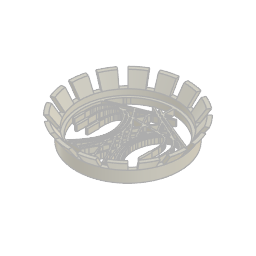
tree-aperture-v10 (Autodesk Fusion 360 design; units mm, degrees)
Autodesk Fusion 360 part; units mm, degrees
(part 1 of 3)
sketch "Sketch1" plane through (0, 0, 0) normal (0, 0, 1) x (1, 0, 0)
  line L0 (24.379, -0.087) -> (23.062, -0.162)
  line L1 (23.062, -0.162) -> (21.745, -0.311)
  line L2 (21.745, -0.311) -> (20.577, -0.509)
  line L3 (20.577, -0.509) -> (19.433, -0.758)
  line L4 (19.433, -0.758) -> (18.067, -1.131)
  line L5 (18.067, -1.131) -> (17.097, -1.454)
  line L6 (17.097, -1.454) -> (16.103, -1.827)
  line L7 (16.103, -1.827) -> (14.886, -2.348)
  line L8 (14.886, -2.348) -> (13.618, -2.97)
  line L9 (13.618, -2.97) -> (12.724, -3.467)
  line L10 (12.724, -3.467) -> (11.705, -4.088)
  line L11 (11.705, -4.088) -> (10.686, -4.784)
  line L12 (10.686, -4.784) -> (9.891, -5.38)
  line L13 (9.891, -5.38) -> (8.574, -6.474)
  line L14 (8.574, -6.474) -> (6.809, -8.188)
  line L15 (6.809, -8.188) -> (5.939, -9.158)
  line L16 (5.939, -9.158) -> (5.244, -10.002)
  line L17 (5.244, -10.002) -> (4.573, -10.897)
  line L18 (4.573, -10.897) -> (3.877, -11.916)
  line L19 (3.877, -11.916) -> (3.231, -12.96)
  line L20 (3.231, -12.96) -> (2.659, -14.003)
  line L21 (2.659, -14.003) -> (2.212, -14.923)
  line L22 (2.212, -14.923) -> (1.764, -15.967)
  line L23 (1.764, -15.967) -> (1.441, -16.812)
  line L24 (1.441, -16.812) -> (0.919, -18.427)
  line L25 (0.919, -18.427) -> (0.547, -19.868)
  line L26 (0.547, -19.868) -> (0.348, -20.862)
  line L27 (0.348, -20.862) -> (0.149, -22.229)
  line L28 (0.149, -22.229) -> (0.025, -23.521)
  line L29 (0.025, -23.521) -> (0, -25.957)
  line L30 (0, -25.957) -> (0.149, -27.87)
  line L31 (0.149, -27.87) -> (0.298, -28.889)
  line L32 (0.298, -28.889) -> (0.596, -30.355)
  line L33 (0.596, -30.355) -> (0.944, -31.672)
  line L34 (0.944, -31.672) -> (1.367, -32.99)
  line L35 (1.367, -32.99) -> (2.137, -34.903)
  line L36 (2.137, -34.903) -> (2.783, -36.22)
  line L37 (2.783, -36.22) -> (3.355, -37.239)
  line L38 (3.355, -37.239) -> (4.647, -39.202)
  line L39 (4.647, -39.202) -> (5.666, -40.519)
  line L40 (5.666, -40.519) -> (6.287, -41.24)
  line L41 (6.287, -41.24) -> (7.828, -42.831)
  line L42 (7.828, -42.831) -> (8.921, -43.8)
  line L43 (8.921, -43.8) -> (10.04, -44.694)
  line L44 (10.04, -44.694) -> (12.003, -46.036)
  line L45 (12.003, -46.036) -> (13.917, -47.13)
  line L46 (13.917, -47.13) -> (15.084, -47.701)
  line L47 (15.084, -47.701) -> (16.327, -48.223)
  line L48 (16.327, -48.223) -> (17.57, -48.67)
  line L49 (17.57, -48.67) -> (18.539, -48.969)
  line L50 (18.539, -48.969) -> (19.906, -49.317)
  line L51 (19.906, -49.317) -> (21.645, -49.64)
  line L52 (21.645, -49.64) -> (21.844, -49.64)
  line L53 (21.844, -49.64) -> (21.993, -49.689)
  line L54 (21.993, -49.689) -> (22.913, -49.789)
  line L55 (22.913, -49.789) -> (24.105, -49.863)
  line L56 (24.105, -49.863) -> (25.323, -49.888)
  line L57 (25.323, -49.888) -> (26.566, -49.838)
  line L58 (26.566, -49.838) -> (28.032, -49.689)
  line L59 (28.032, -49.689) -> (29.125, -49.515)
  line L60 (29.125, -49.515) -> (30.442, -49.242)
  line L61 (30.442, -49.242) -> (31.834, -48.869)
  line L62 (31.834, -48.869) -> (33.052, -48.472)
  line L63 (33.052, -48.472) -> (34.046, -48.099)
  line L64 (34.046, -48.099) -> (35.089, -47.652)
  line L65 (35.089, -47.652) -> (36.158, -47.13)
  line L66 (36.158, -47.13) -> (37.251, -46.533)
  line L67 (37.251, -46.533) -> (38.593, -45.713)
  line L68 (38.593, -45.713) -> (40.383, -44.446)
  line L69 (40.383, -44.446) -> (41.277, -43.725)
  line L70 (41.277, -43.725) -> (42.147, -42.955)
  line L71 (42.147, -42.955) -> (43.067, -42.06)
  line L72 (43.067, -42.06) -> (44.21, -40.793)
  line L73 (44.21, -40.793) -> (44.806, -40.047)
  line L74 (44.806, -40.047) -> (46.123, -38.159)
  line L75 (46.123, -38.159) -> (46.794, -37.04)
  line L76 (46.794, -37.04) -> (47.316, -36.071)
  line L77 (47.316, -36.071) -> (47.763, -35.152)
  line L78 (47.763, -35.152) -> (48.385, -33.685)
  line L79 (48.385, -33.685) -> (48.708, -32.791)
  line L80 (48.708, -32.791) -> (49.155, -31.325)
  line L81 (49.155, -31.325) -> (49.478, -30.007)
  line L82 (49.478, -30.007) -> (49.677, -28.939)
  line L83 (49.677, -28.939) -> (49.925, -26.802)
  line L84 (49.925, -26.802) -> (49.975, -25.882)
  line L85 (49.975, -25.882) -> (49.975, -24.093)
  line L86 (49.975, -24.093) -> (49.801, -22.005)
  line L87 (49.801, -22.005) -> (49.602, -20.738)
  line L88 (49.602, -20.738) -> (49.354, -19.545)
  line L89 (49.354, -19.545) -> (48.981, -18.154)
  line L90 (48.981, -18.154) -> (48.534, -16.787)
  line L91 (48.534, -16.787) -> (48.136, -15.768)
  line L92 (48.136, -15.768) -> (47.689, -14.774)
  line L93 (47.689, -14.774) -> (46.72, -12.935)
  line L94 (46.72, -12.935) -> (45.403, -10.897)
  line L95 (45.403, -10.897) -> (44.483, -9.679)
  line L96 (44.483, -9.679) -> (43.713, -8.76)
  line L97 (43.713, -8.76) -> (42.122, -7.095)
  line L98 (42.122, -7.095) -> (40.905, -6.001)
  line L99 (40.905, -6.001) -> (39.811, -5.132)
  line L100 (39.811, -5.132) -> (38.917, -4.486)
  line L101 (38.917, -4.486) -> (37.898, -3.815)
  line L102 (37.898, -3.815) -> (36.705, -3.119)
  line L103 (36.705, -3.119) -> (35.611, -2.547)
  line L104 (35.611, -2.547) -> (33.673, -1.702)
  line L105 (33.673, -1.702) -> (31.436, -0.957)
  line L106 (31.436, -0.957) -> (30.169, -0.634)
  line L107 (30.169, -0.634) -> (29.175, -0.435)
  line L108 (29.175, -0.435) -> (27.833, -0.236)
  line L109 (27.833, -0.236) -> (26.491, -0.112)
  line L110 (26.491, -0.112) -> (24.379, -0.087)
  line L111 (10.934, -5.529) -> (12.202, -4.66)
  line L112 (12.202, -4.66) -> (12.972, -4.187)
  line L113 (12.972, -4.187) -> (14.14, -3.541)
  line L114 (14.14, -3.541) -> (15.209, -3.019)
  line L115 (15.209, -3.019) -> (17.222, -2.199)
  line L116 (17.222, -2.199) -> (18.191, -1.876)
  line L117 (18.191, -1.876) -> (18.29, -1.876)
  line L118 (18.29, -1.876) -> (18.613, -1.752)
  line L119 (18.613, -1.752) -> (19.831, -1.429)
  line L120 (19.831, -1.429) -> (21.074, -1.18)
  line L121 (21.074, -1.18) -> (22.44, -0.982)
  line L122 (22.44, -0.982) -> (24.503, -0.833)
  line L123 (24.503, -0.833) -> (26.417, -0.857)
  line L124 (26.417, -0.857) -> (26.715, -0.907)
  line L125 (26.715, -0.907) -> (27.361, -0.932)
  line L126 (27.361, -0.932) -> (28.678, -1.106)
  line L127 (28.678, -1.106) -> (29.771, -1.305)
  line L128 (29.771, -1.305) -> (29.871, -1.354)
  line L129 (29.871, -1.354) -> (29.995, -1.354)
  line L130 (29.995, -1.354) -> (30.815, -1.553)
  line L131 (30.815, -1.553) -> (31.933, -1.876)
  line L132 (31.933, -1.876) -> (33.077, -2.274)
  line L133 (33.077, -2.274) -> (34.965, -3.069)
  line L134 (34.965, -3.069) -> (36.332, -3.765)
  line L135 (36.332, -3.765) -> (37.401, -4.386)
  line L136 (37.401, -4.386) -> (38.32, -4.983)
  line L137 (38.32, -4.983) -> (39.389, -5.753)
  line L138 (39.389, -5.753) -> (40.184, -6.374)
  line L139 (40.184, -6.374) -> (41.153, -7.219)
  line L140 (41.153, -7.219) -> (42.893, -8.959)
  line L141 (42.893, -8.959) -> (43.588, -9.754)
  line L142 (43.588, -9.754) -> (44.508, -10.922)
  line L143 (44.508, -10.922) -> (45.452, -12.289)
  line L144 (45.452, -12.289) -> (45.999, -13.183)
  line L145 (45.999, -13.183) -> (46.571, -14.202)
  line L146 (46.571, -14.202) -> (47.068, -15.196)
  line L147 (47.068, -15.196) -> (47.838, -17.035)
  line L148 (47.838, -17.035) -> (48.236, -18.228)
  line L149 (48.236, -18.228) -> (48.559, -19.396)
  line L150 (48.559, -19.396) -> (48.807, -20.49)
  line L151 (48.807, -20.49) -> (49.006, -21.608)
  line L152 (49.006, -21.608) -> (49.13, -22.527)
  line L153 (49.13, -22.527) -> (49.254, -24.267)
  line L154 (49.254, -24.267) -> (49.254, -25.584)
  line L155 (49.254, -25.584) -> (49.205, -26.628)
  line L156 (49.205, -26.628) -> (49.006, -28.467)
  line L157 (49.006, -28.467) -> (48.559, -30.703)
  line L158 (48.559, -30.703) -> (48.236, -31.846)
  line L159 (48.236, -31.846) -> (47.788, -33.164)
  line L160 (47.788, -33.164) -> (46.943, -35.152)
  line L161 (46.943, -35.152) -> (46.248, -36.518)
  line L162 (46.248, -36.518) -> (45.651, -37.537)
  line L163 (45.651, -37.537) -> (44.359, -39.426)
  line L164 (44.359, -39.426) -> (43.539, -40.445)
  line L165 (43.539, -40.445) -> (42.893, -41.166)
  line L166 (42.893, -41.166) -> (42.172, -41.911)
  line L167 (42.172, -41.911) -> (41.153, -42.855)
  line L168 (41.153, -42.855) -> (39.488, -44.197)
  line L169 (39.488, -44.197) -> (39.364, -44.247)
  line L170 (39.364, -44.247) -> (39.165, -44.048)
  line L171 (39.165, -44.048) -> (37.798, -42.458)
  line L172 (37.798, -42.458) -> (36.481, -40.842)
  line L173 (36.481, -40.842) -> (35.065, -38.904)
  line L174 (35.065, -38.904) -> (33.847, -37.09)
  line L175 (33.847, -37.09) -> (33.151, -35.922)
  line L176 (33.151, -35.922) -> (32.43, -34.53)
  line L177 (32.43, -34.53) -> (31.884, -33.213)
  line L178 (31.884, -33.213) -> (31.486, -31.971)
  line L179 (31.486, -31.971) -> (31.238, -30.902)
  line L180 (31.238, -30.902) -> (31.088, -29.908)
  line L181 (31.088, -29.908) -> (30.989, -28.442)
  line L182 (30.989, -28.442) -> (31.039, -26.951)
  line L183 (31.039, -26.951) -> (31.163, -25.932)
  line L184 (31.163, -25.932) -> (31.486, -24.317)
  line L185 (31.486, -24.317) -> (31.884, -22.975)
  line L186 (31.884, -22.975) -> (32.306, -21.856)
  line L187 (32.306, -21.856) -> (32.878, -20.614)
  line L188 (32.878, -20.614) -> (33.524, -19.471)
  line L189 (33.524, -19.471) -> (34.418, -18.203)
  line L190 (34.418, -18.203) -> (34.866, -17.681)
  line L191 (34.866, -17.681) -> (35.661, -16.911)
  line L192 (35.661, -16.911) -> (35.835, -16.936)
  line L193 (35.835, -16.936) -> (36.332, -17.259)
  line L194 (36.332, -17.259) -> (37.028, -17.955)
  line L195 (37.028, -17.955) -> (37.525, -18.725)
  line L196 (37.525, -18.725) -> (37.724, -19.123)
  line L197 (37.724, -19.123) -> (38.047, -19.943)
  line L198 (38.047, -19.943) -> (38.37, -21.185)
  line L199 (38.37, -21.185) -> (38.494, -21.956)
  line L200 (38.494, -21.956) -> (38.593, -23.149)
  line L201 (38.593, -23.149) -> (38.593, -26.628)
  line L202 (38.593, -26.628) -> (38.544, -26.677)
  line L203 (38.544, -26.677) -> (38.419, -26.702)
  line L204 (38.419, -26.702) -> (38.345, -26.827)
  line L205 (38.345, -26.827) -> (38.345, -33.014)
  line L206 (38.345, -33.014) -> (38.469, -33.139)
  line L207 (38.469, -33.139) -> (39.438, -33.114)
  line L208 (39.438, -33.114) -> (39.538, -32.99)
  line L209 (39.538, -32.99) -> (39.538, -26.851)
  line L210 (39.538, -26.851) -> (39.438, -26.702)
  line L211 (39.438, -26.702) -> (39.289, -26.628)
  line L212 (39.289, -26.628) -> (39.289, -22.975)
  line L213 (39.289, -22.975) -> (39.115, -21.334)
  line L214 (39.115, -21.334) -> (38.991, -20.688)
  line L215 (38.991, -20.688) -> (38.792, -19.943)
  line L216 (38.792, -19.943) -> (38.593, -19.346)
  line L217 (38.593, -19.346) -> (38.196, -18.452)
  line L218 (38.196, -18.452) -> (37.898, -17.93)
  line L219 (37.898, -17.93) -> (37.5, -17.383)
  line L220 (37.5, -17.383) -> (37.053, -16.911)
  line L221 (37.053, -16.911) -> (36.506, -16.513)
  line L222 (36.506, -16.513) -> (36.407, -16.414)
  line L223 (36.407, -16.414) -> (36.407, -16.364)
  line L224 (36.407, -16.364) -> (36.754, -16.116)
  line L225 (36.754, -16.116) -> (37.475, -15.743)
  line L226 (37.475, -15.743) -> (38.221, -15.47)
  line L227 (38.221, -15.47) -> (38.345, -15.47)
  line L228 (38.345, -15.47) -> (39.24, -15.867)
  line L229 (39.24, -15.867) -> (39.911, -16.29)
  line L230 (39.911, -16.29) -> (40.432, -16.712)
  line L231 (40.432, -16.712) -> (41.252, -17.582)
  line L232 (41.252, -17.582) -> (41.625, -18.104)
  line L233 (41.625, -18.104) -> (41.998, -18.75)
  line L234 (41.998, -18.75) -> (42.271, -19.322)
  line L235 (42.271, -19.322) -> (42.57, -20.092)
  line L236 (42.57, -20.092) -> (42.917, -21.434)
  line L237 (42.917, -21.434) -> (43.042, -22.229)
  line L238 (43.042, -22.229) -> (43.116, -23.149)
  line L239 (43.116, -23.149) -> (43.116, -28.119)
  line L240 (43.116, -28.119) -> (42.942, -28.168)
  line L241 (42.942, -28.168) -> (42.843, -28.342)
  line L242 (42.843, -28.342) -> (42.843, -34.257)
  line L243 (42.843, -34.257) -> (42.967, -34.406)
  line L244 (42.967, -34.406) -> (43.887, -34.406)
  line L245 (43.887, -34.406) -> (44.011, -34.282)
  line L246 (44.011, -34.282) -> (44.011, -28.268)
  line L247 (44.011, -28.268) -> (43.936, -28.168)
  line L248 (43.936, -28.168) -> (43.837, -28.119)
  line L249 (43.837, -28.119) -> (43.837, -23.323)
  line L250 (43.837, -23.323) -> (43.762, -22.279)
  line L251 (43.762, -22.279) -> (43.564, -21.061)
  line L252 (43.564, -21.061) -> (43.315, -20.092)
  line L253 (43.315, -20.092) -> (42.942, -19.073)
  line L254 (42.942, -19.073) -> (42.57, -18.303)
  line L255 (42.57, -18.303) -> (42.172, -17.632)
  line L256 (42.172, -17.632) -> (41.799, -17.11)
  line L257 (41.799, -17.11) -> (41.153, -16.389)
  line L258 (41.153, -16.389) -> (40.383, -15.743)
  line L259 (40.383, -15.743) -> (39.712, -15.321)
  line L260 (39.712, -15.321) -> (39.687, -15.246)
  line L261 (39.687, -15.246) -> (39.761, -15.196)
  line L262 (39.761, -15.196) -> (40.532, -15.221)
  line L263 (40.532, -15.221) -> (41.079, -15.296)
  line L264 (41.079, -15.296) -> (41.6, -15.42)
  line L265 (41.6, -15.42) -> (42.545, -15.793)
  line L266 (42.545, -15.793) -> (43.191, -16.166)
  line L267 (43.191, -16.166) -> (43.837, -16.663)
  line L268 (43.837, -16.663) -> (44.409, -17.234)
  line L269 (44.409, -17.234) -> (44.756, -17.657)
  line L270 (44.756, -17.657) -> (45.353, -18.576)
  line L271 (45.353, -18.576) -> (45.8, -19.496)
  line L272 (45.8, -19.496) -> (46.123, -20.365)
  line L273 (46.123, -20.365) -> (46.347, -21.161)
  line L274 (46.347, -21.161) -> (46.496, -21.906)
  line L275 (46.496, -21.906) -> (46.62, -22.95)
  line L276 (46.62, -22.95) -> (46.645, -26.205)
  line L277 (46.645, -26.205) -> (46.546, -26.28)
  line L278 (46.546, -26.28) -> (46.496, -26.379)
  line L279 (46.496, -26.379) -> (46.496, -31.747)
  line L280 (46.496, -31.747) -> (46.67, -31.871)
  line L281 (46.67, -31.871) -> (47.515, -31.846)
  line L282 (47.515, -31.846) -> (47.614, -31.722)
  line L283 (47.614, -31.722) -> (47.614, -26.379)
  line L284 (47.614, -26.379) -> (47.54, -26.255)
  line L285 (47.54, -26.255) -> (47.416, -26.23)
  line L286 (47.416, -26.23) -> (47.366, -26.18)
  line L287 (47.366, -26.18) -> (47.366, -23.621)
  line L288 (47.366, -23.621) -> (47.316, -22.826)
  line L289 (47.316, -22.826) -> (47.117, -21.384)
  line L290 (47.117, -21.384) -> (46.918, -20.539)
  line L291 (46.918, -20.539) -> (46.67, -19.744)
  line L292 (46.67, -19.744) -> (46.372, -18.999)
  line L293 (46.372, -18.999) -> (45.9, -18.079)
  line L294 (45.9, -18.079) -> (45.452, -17.383)
  line L295 (45.452, -17.383) -> (45.005, -16.812)
  line L296 (45.005, -16.812) -> (44.483, -16.265)
  line L297 (44.483, -16.265) -> (43.862, -15.743)
  line L298 (43.862, -15.743) -> (42.843, -15.122)
  line L299 (42.843, -15.122) -> (41.725, -14.699)
  line L300 (41.725, -14.699) -> (41.054, -14.55)
  line L301 (41.054, -14.55) -> (40.507, -14.476)
  line L302 (40.507, -14.476) -> (39.563, -14.426)
  line L303 (39.563, -14.426) -> (38.792, -14.327)
  line L304 (38.792, -14.327) -> (34.816, -12.463)
  line L305 (34.816, -12.463) -> (34.766, -12.363)
  line L306 (34.766, -12.363) -> (35.313, -11.618)
  line L307 (35.313, -11.618) -> (35.437, -11.593)
  line L308 (35.437, -11.593) -> (38.917, -13.009)
  line L309 (38.917, -13.009) -> (42.371, -14.476)
  line L310 (42.371, -14.476) -> (42.445, -14.476)
  line L311 (42.445, -14.476) -> (42.669, -13.954)
  line L312 (42.669, -13.954) -> (42.719, -13.705)
  line L313 (42.719, -13.705) -> (39.19, -12.239)
  line L314 (39.19, -12.239) -> (37.351, -11.518)
  line L315 (37.351, -11.518) -> (36.332, -11.071)
  line L316 (36.332, -11.071) -> (35.288, -10.673)
  line L317 (35.288, -10.673) -> (32.58, -9.53)
  line L318 (32.58, -9.53) -> (32.505, -9.53)
  line L319 (32.505, -9.53) -> (31.958, -9.282)
  line L320 (31.958, -9.282) -> (31.585, -9.158)
  line L321 (31.585, -9.158) -> (28.38, -7.791)
  line L322 (28.38, -7.791) -> (27.883, -7.542)
  line L323 (27.883, -7.542) -> (27.908, -7.468)
  line L324 (27.908, -7.468) -> (31.262, -5.852)
  line L325 (31.262, -5.852) -> (31.312, -5.803)
  line L326 (31.312, -5.803) -> (31.312, -5.728)
  line L327 (31.312, -5.728) -> (30.989, -5.057)
  line L328 (30.989, -5.057) -> (30.915, -5.057)
  line L329 (30.915, -5.057) -> (27.038, -7.02)
  line L330 (27.038, -7.02) -> (26.789, -7.07)
  line L331 (26.789, -7.07) -> (26.069, -6.722)
  line L332 (26.069, -6.722) -> (26.044, -6.623)
  line L333 (26.044, -6.623) -> (28.33, -5.455)
  line L334 (28.33, -5.455) -> (28.355, -5.331)
  line L335 (28.355, -5.331) -> (28.032, -4.684)
  line L336 (28.032, -4.684) -> (27.336, -5.007)
  line L337 (27.336, -5.007) -> (25.075, -6.2)
  line L338 (25.075, -6.2) -> (24.975, -6.2)
  line L339 (24.975, -6.2) -> (22.639, -4.983)
  line L340 (22.639, -4.983) -> (21.993, -4.684)
  line L341 (21.993, -4.684) -> (21.645, -5.355)
  line L342 (21.645, -5.355) -> (21.695, -5.455)
  line L343 (21.695, -5.455) -> (24.006, -6.623)
  line L344 (24.006, -6.623) -> (23.981, -6.722)
  line L345 (23.981, -6.722) -> (23.236, -7.095)
  line L346 (23.236, -7.095) -> (22.913, -6.971)
  line L347 (22.913, -6.971) -> (19.135, -5.082)
  line L348 (19.135, -5.082) -> (19.036, -5.082)
  line L349 (19.036, -5.082) -> (18.738, -5.678)
  line L350 (18.738, -5.678) -> (18.713, -5.803)
  line L351 (18.713, -5.803) -> (18.762, -5.852)
  line L352 (18.762, -5.852) -> (22.142, -7.468)
  line L353 (22.142, -7.468) -> (22.167, -7.567)
  line L354 (22.167, -7.567) -> (18.588, -9.133)
  line L355 (18.588, -9.133) -> (12.351, -11.643)
  line L356 (12.351, -11.643) -> (7.306, -13.73)
  line L357 (7.306, -13.73) -> (7.331, -13.904)
  line L358 (7.331, -13.904) -> (7.58, -14.476)
  line L359 (7.58, -14.476) -> (7.654, -14.476)
  line L360 (7.654, -14.476) -> (14.612, -11.593)
  line L361 (14.612, -11.593) -> (14.687, -11.593)
  line L362 (14.687, -11.593) -> (14.786, -11.692)
  line L363 (14.786, -11.692) -> (15.234, -12.338)
  line L364 (15.234, -12.338) -> (15.283, -12.363)
  line L365 (15.283, -12.363) -> (15.283, -12.413)
  line L366 (15.283, -12.413) -> (15.184, -12.488)
  line L367 (15.184, -12.488) -> (11.257, -14.327)
  line L368 (11.257, -14.327) -> (10.736, -14.401)
  line L369 (10.736, -14.401) -> (9.568, -14.476)
  line L370 (9.568, -14.476) -> (8.822, -14.6)
  line L371 (8.822, -14.6) -> (7.878, -14.873)
  line L372 (7.878, -14.873) -> (6.909, -15.321)
  line L373 (6.909, -15.321) -> (6.064, -15.867)
  line L374 (6.064, -15.867) -> (5.442, -16.389)
  line L375 (5.442, -16.389) -> (4.722, -17.16)
  line L376 (4.722, -17.16) -> (4.125, -18.004)
  line L377 (4.125, -18.004) -> (3.628, -18.949)
  line L378 (3.628, -18.949) -> (3.28, -19.794)
  line L379 (3.28, -19.794) -> (2.908, -21.061)
  line L380 (2.908, -21.061) -> (2.709, -22.229)
  line L381 (2.709, -22.229) -> (2.609, -23.397)
  line L382 (2.609, -23.397) -> (2.609, -26.18)
  line L383 (2.609, -26.18) -> (2.46, -26.255)
  line L384 (2.46, -26.255) -> (2.386, -26.379)
  line L385 (2.386, -26.379) -> (2.411, -31.772)
  line L386 (2.411, -31.772) -> (2.56, -31.871)
  line L387 (2.56, -31.871) -> (3.429, -31.846)
  line L388 (3.429, -31.846) -> (3.529, -31.747)
  line L389 (3.529, -31.747) -> (3.529, -26.354)
  line L390 (3.529, -26.354) -> (3.454, -26.255)
  line L391 (3.454, -26.255) -> (3.305, -26.18)
  line L392 (3.305, -26.18) -> (3.33, -23.298)
  line L393 (3.33, -23.298) -> (3.405, -22.403)
  line L394 (3.405, -22.403) -> (3.529, -21.608)
  line L395 (3.529, -21.608) -> (3.802, -20.539)
  line L396 (3.802, -20.539) -> (4.15, -19.57)
  line L397 (4.15, -19.57) -> (4.548, -18.75)
  line L398 (4.548, -18.75) -> (5.119, -17.855)
  line L399 (5.119, -17.855) -> (5.567, -17.309)
  line L400 (5.567, -17.309) -> (6.362, -16.563)
  line L401 (6.362, -16.563) -> (7.083, -16.066)
  line L402 (7.083, -16.066) -> (7.853, -15.668)
  line L403 (7.853, -15.668) -> (8.549, -15.42)
  line L404 (8.549, -15.42) -> (9.493, -15.221)
  line L405 (9.493, -15.221) -> (10.437, -15.196)
  line L406 (10.437, -15.196) -> (10.487, -15.296)
  line L407 (10.487, -15.296) -> (9.965, -15.619)
  line L408 (9.965, -15.619) -> (9.195, -16.215)
  line L409 (9.195, -16.215) -> (8.499, -16.911)
  line L410 (8.499, -16.911) -> (7.977, -17.582)
  line L411 (7.977, -17.582) -> (7.455, -18.427)
  line L412 (7.455, -18.427) -> (7.083, -19.197)
  line L413 (7.083, -19.197) -> (6.759, -20.067)
  line L414 (6.759, -20.067) -> (6.436, -21.334)
  line L415 (6.436, -21.334) -> (6.312, -22.105)
  line L416 (6.312, -22.105) -> (6.213, -23.173)
  line L417 (6.213, -23.173) -> (6.213, -28.019)
  line L418 (6.213, -28.019) -> (6.188, -28.119)
  line L419 (6.188, -28.119) -> (6.039, -28.268)
  line L420 (6.039, -28.268) -> (6.039, -34.307)
  line L421 (6.039, -34.307) -> (6.163, -34.406)
  line L422 (6.163, -34.406) -> (7.058, -34.406)
  line L423 (7.058, -34.406) -> (7.182, -34.282)
  line L424 (7.182, -34.282) -> (7.182, -28.268)
  line L425 (7.182, -28.268) -> (7.058, -28.144)
  line L426 (7.058, -28.144) -> (6.958, -28.144)
  line L427 (6.958, -28.144) -> (6.909, -28.094)
  line L428 (6.909, -28.094) -> (6.909, -23.571)
  line L429 (6.909, -23.571) -> (6.983, -22.478)
  line L430 (6.983, -22.478) -> (7.058, -21.956)
  line L431 (7.058, -21.956) -> (7.381, -20.514)
  line L432 (7.381, -20.514) -> (7.629, -19.794)
  line L433 (7.629, -19.794) -> (8.077, -18.825)
  line L434 (8.077, -18.825) -> (8.499, -18.129)
  line L435 (8.499, -18.129) -> (9.046, -17.408)
  line L436 (9.046, -17.408) -> (9.717, -16.737)
  line L437 (9.717, -16.737) -> (10.288, -16.29)
  line L438 (10.288, -16.29) -> (11.108, -15.793)
  line L439 (11.108, -15.793) -> (11.655, -15.544)
  line L440 (11.655, -15.544) -> (11.953, -15.495)
  line L441 (11.953, -15.495) -> (12.525, -15.718)
  line L442 (12.525, -15.718) -> (13.37, -16.166)
  line L443 (13.37, -16.166) -> (13.593, -16.315)
  line L444 (13.593, -16.315) -> (13.643, -16.414)
  line L445 (13.643, -16.414) -> (13.121, -16.787)
  line L446 (13.121, -16.787) -> (12.724, -17.16)
  line L447 (12.724, -17.16) -> (12.401, -17.532)
  line L448 (12.401, -17.532) -> (11.978, -18.154)
  line L449 (11.978, -18.154) -> (11.754, -18.551)
  line L450 (11.754, -18.551) -> (11.307, -19.595)
  line L451 (11.307, -19.595) -> (11.059, -20.415)
  line L452 (11.059, -20.415) -> (10.91, -21.061)
  line L453 (10.91, -21.061) -> (10.785, -21.807)
  line L454 (10.785, -21.807) -> (10.661, -23.248)
  line L455 (10.661, -23.248) -> (10.686, -26.379)
  line L456 (10.686, -26.379) -> (10.661, -26.653)
  line L457 (10.661, -26.653) -> (10.562, -26.702)
  line L458 (10.562, -26.702) -> (10.462, -26.827)
  line L459 (10.462, -26.827) -> (10.487, -33.064)
  line L460 (10.487, -33.064) -> (10.586, -33.139)
  line L461 (10.586, -33.139) -> (11.506, -33.139)
  line L462 (11.506, -33.139) -> (11.605, -33.064)
  line L463 (11.605, -33.064) -> (11.63, -32.99)
  line L464 (11.63, -32.99) -> (11.63, -26.827)
  line L465 (11.63, -26.827) -> (11.531, -26.702)
  line L466 (11.531, -26.702) -> (11.407, -26.677)
  line L467 (11.407, -26.677) -> (11.357, -26.628)
  line L468 (11.357, -26.628) -> (11.357, -23.646)
  line L469 (11.357, -23.646) -> (11.481, -22.03)
  line L470 (11.481, -22.03) -> (11.655, -21.036)
  line L471 (11.655, -21.036) -> (12.003, -19.794)
  line L472 (12.003, -19.794) -> (12.251, -19.197)
  line L473 (12.251, -19.197) -> (12.649, -18.452)
  line L474 (12.649, -18.452) -> (13.022, -17.93)
  line L475 (13.022, -17.93) -> (13.469, -17.458)
  line L476 (13.469, -17.458) -> (13.743, -17.234)
  line L477 (13.743, -17.234) -> (14.314, -16.886)
  line L478 (14.314, -16.886) -> (14.364, -16.886)
  line L479 (14.364, -16.886) -> (15.283, -17.806)
  line L480 (15.283, -17.806) -> (15.656, -18.253)
  line L481 (15.656, -18.253) -> (16.352, -19.222)
  line L482 (16.352, -19.222) -> (16.923, -20.167)
  line L483 (16.923, -20.167) -> (17.321, -20.937)
  line L484 (17.321, -20.937) -> (18.017, -22.577)
  line L485 (18.017, -22.577) -> (18.489, -24.043)
  line L486 (18.489, -24.043) -> (18.688, -24.838)
  line L487 (18.688, -24.838) -> (18.887, -25.932)
  line L488 (18.887, -25.932) -> (19.036, -27.547)
  line L489 (19.036, -27.547) -> (19.011, -29.386)
  line L490 (19.011, -29.386) -> (18.812, -30.877)
  line L491 (18.812, -30.877) -> (18.415, -32.468)
  line L492 (18.415, -32.468) -> (18.216, -33.064)
  line L493 (18.216, -33.064) -> (17.52, -34.704)
  line L494 (17.52, -34.704) -> (16.874, -35.922)
  line L495 (16.874, -35.922) -> (15.979, -37.413)
  line L496 (15.979, -37.413) -> (14.314, -39.824)
  line L497 (14.314, -39.824) -> (12.798, -41.762)
  line L498 (12.798, -41.762) -> (10.711, -44.197)
  line L499 (10.711, -44.197) -> (10.586, -44.172)
  line L500 (10.586, -44.172) -> (9.568, -43.377)
  line L501 (9.568, -43.377) -> (8.822, -42.731)
  line L502 (8.822, -42.731) -> (7.803, -41.762)
  line L503 (7.803, -41.762) -> (6.387, -40.221)
  line L504 (6.387, -40.221) -> (5.318, -38.854)
  line L505 (5.318, -38.854) -> (4.871, -38.233)
  line L506 (4.871, -38.233) -> (4.1, -37.04)
  line L507 (4.1, -37.04) -> (3.504, -35.997)
  line L508 (3.504, -35.997) -> (2.858, -34.704)
  line L509 (2.858, -34.704) -> (2.435, -33.735)
  line L510 (2.435, -33.735) -> (1.914, -32.319)
  line L511 (1.914, -32.319) -> (1.342, -30.331)
  line L512 (1.342, -30.331) -> (1.093, -29.163)
  line L513 (1.093, -29.163) -> (0.944, -28.069)
  line L514 (0.944, -28.069) -> (0.895, -27.92)
  line L515 (0.895, -27.92) -> (0.77, -26.727)
  line L516 (0.77, -26.727) -> (0.721, -25.708)
  line L517 (0.721, -25.708) -> (0.77, -23.447)
  line L518 (0.77, -23.447) -> (0.845, -22.577)
  line L519 (0.845, -22.577) -> (1.019, -21.31)
  line L520 (1.019, -21.31) -> (1.292, -19.968)
  line L521 (1.292, -19.968) -> (1.342, -19.868)
  line L522 (1.342, -19.868) -> (1.342, -19.744)
  line L523 (1.342, -19.744) -> (1.789, -18.129)
  line L524 (1.789, -18.129) -> (2.361, -16.489)
  line L525 (2.361, -16.489) -> (2.883, -15.246)
  line L526 (2.883, -15.246) -> (3.454, -14.103)
  line L527 (3.454, -14.103) -> (4.498, -12.338)
  line L528 (4.498, -12.338) -> (4.995, -11.593)
  line L529 (4.995, -11.593) -> (5.765, -10.549)
  line L530 (5.765, -10.549) -> (7.381, -8.685)
  line L531 (7.381, -8.685) -> (8.946, -7.145)
  line L532 (8.946, -7.145) -> (9.667, -6.523)
  line L533 (9.667, -6.523) -> (10.934, -5.529)
  line L534 (11.009, -44.421) -> (19.21, -44.396)
  line L535 (19.21, -44.396) -> (19.284, -44.322)
  line L536 (19.284, -44.322) -> (19.856, -42.806)
  line L537 (19.856, -42.806) -> (20.577, -41.339)
  line L538 (20.577, -41.339) -> (22.44, -38.059)
  line L539 (22.44, -38.059) -> (22.763, -37.562)
  line L540 (22.763, -37.562) -> (22.763, -37.512)
  line L541 (22.763, -37.512) -> (22.838, -37.488)
  line L542 (22.838, -37.488) -> (23.285, -38.68)
  line L543 (23.285, -38.68) -> (23.36, -38.979)
  line L544 (23.36, -38.979) -> (24.627, -42.582)
  line L545 (24.627, -42.582) -> (24.578, -42.88)
  line L546 (24.578, -42.88) -> (24.453, -43.154)
  line L547 (24.453, -43.154) -> (24.105, -44.222)
  line L548 (24.105, -44.222) -> (24.105, -44.322)
  line L549 (24.105, -44.322) -> (24.18, -44.396)
  line L550 (24.18, -44.396) -> (25.82, -44.396)
  line L551 (25.82, -44.396) -> (25.895, -44.322)
  line L552 (25.895, -44.322) -> (25.895, -44.197)
  line L553 (25.895, -44.197) -> (25.373, -42.731)
  line L554 (25.373, -42.731) -> (25.373, -42.557)
  line L555 (25.373, -42.557) -> (26.044, -40.619)
  line L556 (26.044, -40.619) -> (26.143, -40.42)
  line L557 (26.143, -40.42) -> (26.466, -39.376)
  line L558 (26.466, -39.376) -> (26.864, -38.333)
  line L559 (26.864, -38.333) -> (27.112, -37.537)
  line L560 (27.112, -37.537) -> (27.187, -37.512)
  line L561 (27.187, -37.512) -> (27.584, -38.159)
  line L562 (27.584, -38.159) -> (29.125, -40.942)
  line L563 (29.125, -40.942) -> (29.896, -42.532)
  line L564 (29.896, -42.532) -> (30.542, -44.098)
  line L565 (30.542, -44.098) -> (30.591, -44.297)
  line L566 (30.591, -44.297) -> (30.691, -44.396)
  line L567 (30.691, -44.396) -> (39.041, -44.396)
  line L568 (39.041, -44.396) -> (39.066, -44.471)
  line L569 (39.066, -44.471) -> (37.649, -45.44)
  line L570 (37.649, -45.44) -> (36.605, -46.061)
  line L571 (36.605, -46.061) -> (35.388, -46.707)
  line L572 (35.388, -46.707) -> (33.772, -47.428)
  line L573 (33.772, -47.428) -> (32.207, -48)
  line L574 (32.207, -48) -> (30.442, -48.497)
  line L575 (30.442, -48.497) -> (29.175, -48.77)
  line L576 (29.175, -48.77) -> (28.131, -48.944)
  line L577 (28.131, -48.944) -> (25.969, -49.143)
  line L578 (25.969, -49.143) -> (24.13, -49.143)
  line L579 (24.13, -49.143) -> (21.918, -48.944)
  line L580 (21.918, -48.944) -> (20.477, -48.695)
  line L581 (20.477, -48.695) -> (18.514, -48.198)
  line L582 (18.514, -48.198) -> (16.948, -47.676)
  line L583 (16.948, -47.676) -> (15.507, -47.08)
  line L584 (15.507, -47.08) -> (13.618, -46.136)
  line L585 (13.618, -46.136) -> (12.202, -45.291)
  line L586 (12.202, -45.291) -> (11.034, -44.496)
  line L587 (11.034, -44.496) -> (11.009, -44.421)
  line L588 (31.735, -16.513) -> (32.604, -16.513)
  line L589 (32.604, -16.513) -> (32.629, -16.588)
  line L590 (32.629, -16.588) -> (32.281, -17.035)
  line L591 (32.281, -17.035) -> (31.561, -18.178)
  line L592 (31.561, -18.178) -> (30.815, -19.62)
  line L593 (30.815, -19.62) -> (30.442, -20.465)
  line L594 (30.442, -20.465) -> (30.094, -21.359)
  line L595 (30.094, -21.359) -> (29.722, -22.478)
  line L596 (29.722, -22.478) -> (29.25, -24.366)
  line L597 (29.25, -24.366) -> (29.001, -25.957)
  line L598 (29.001, -25.957) -> (28.902, -27.398)
  line L599 (28.902, -27.398) -> (28.926, -29.138)
  line L600 (28.926, -29.138) -> (29.051, -30.331)
  line L601 (29.051, -30.331) -> (29.349, -31.971)
  line L602 (29.349, -31.971) -> (29.771, -33.586)
  line L603 (29.771, -33.586) -> (29.97, -34.207)
  line L604 (29.97, -34.207) -> (30.492, -35.549)
  line L605 (30.492, -35.549) -> (31.064, -36.792)
  line L606 (31.064, -36.792) -> (31.759, -38.109)
  line L607 (31.759, -38.109) -> (32.654, -39.575)
  line L608 (32.654, -39.575) -> (33.971, -41.489)
  line L609 (33.971, -41.489) -> (35.487, -43.452)
  line L610 (35.487, -43.452) -> (35.661, -43.626)
  line L611 (35.661, -43.626) -> (35.636, -43.725)
  line L612 (35.636, -43.725) -> (33.077, -43.725)
  line L613 (33.077, -43.725) -> (33.002, -43.675)
  line L614 (33.002, -43.675) -> (31.809, -41.091)
  line L615 (31.809, -41.091) -> (31.784, -40.967)
  line L616 (31.784, -40.967) -> (31.735, -40.917)
  line L617 (31.735, -40.917) -> (30.268, -37.363)
  line L618 (30.268, -37.363) -> (29.573, -35.475)
  line L619 (29.573, -35.475) -> (28.926, -33.412)
  line L620 (28.926, -33.412) -> (28.628, -32.169)
  line L621 (28.628, -32.169) -> (28.33, -30.554)
  line L622 (28.33, -30.554) -> (28.181, -29.138)
  line L623 (28.181, -29.138) -> (28.156, -27.224)
  line L624 (28.156, -27.224) -> (28.33, -25.186)
  line L625 (28.33, -25.186) -> (28.653, -23.472)
  line L626 (28.653, -23.472) -> (28.951, -22.329)
  line L627 (28.951, -22.329) -> (29.25, -21.434)
  line L628 (29.25, -21.434) -> (29.92, -19.719)
  line L629 (29.92, -19.719) -> (30.517, -18.477)
  line L630 (30.517, -18.477) -> (30.915, -17.756)
  line L631 (30.915, -17.756) -> (31.436, -16.911)
  line L632 (31.436, -16.911) -> (31.735, -16.513)
  line L633 (18.315, -16.513) -> (19.11, -17.756)
  line L634 (19.11, -17.756) -> (20.005, -19.471)
  line L635 (20.005, -19.471) -> (20.775, -21.384)
  line L636 (20.775, -21.384) -> (21.049, -22.204)
  line L637 (21.049, -22.204) -> (21.372, -23.397)
  line L638 (21.372, -23.397) -> (21.695, -25.087)
  line L639 (21.695, -25.087) -> (21.869, -26.876)
  line L640 (21.869, -26.876) -> (21.894, -28.367)
  line L641 (21.894, -28.367) -> (21.745, -30.306)
  line L642 (21.745, -30.306) -> (21.521, -31.648)
  line L643 (21.521, -31.648) -> (21.248, -32.89)
  line L644 (21.248, -32.89) -> (20.85, -34.307)
  line L645 (20.85, -34.307) -> (20.403, -35.649)
  line L646 (20.403, -35.649) -> (19.756, -37.363)
  line L647 (19.756, -37.363) -> (18.738, -39.824)
  line L648 (18.738, -39.824) -> (16.923, -43.651)
  line L649 (16.923, -43.651) -> (16.849, -43.725)
  line L650 (16.849, -43.725) -> (14.513, -43.725)
  line L651 (14.513, -43.725) -> (14.389, -43.675)
  line L652 (14.389, -43.675) -> (14.438, -43.551)
  line L653 (14.438, -43.551) -> (15.134, -42.706)
  line L654 (15.134, -42.706) -> (16.302, -41.141)
  line L655 (16.302, -41.141) -> (17.744, -39.003)
  line L656 (17.744, -39.003) -> (18.564, -37.587)
  line L657 (18.564, -37.587) -> (19.036, -36.667)
  line L658 (19.036, -36.667) -> (19.756, -35.027)
  line L659 (19.756, -35.027) -> (20.303, -33.462)
  line L660 (20.303, -33.462) -> (20.75, -31.697)
  line L661 (20.75, -31.697) -> (20.974, -30.43)
  line L662 (20.974, -30.43) -> (21.123, -28.79)
  line L663 (21.123, -28.79) -> (21.123, -27.15)
  line L664 (21.123, -27.15) -> (21.049, -26.081)
  line L665 (21.049, -26.081) -> (20.85, -24.665)
  line L666 (20.85, -24.665) -> (20.676, -23.844)
  line L667 (20.676, -23.844) -> (20.328, -22.527)
  line L668 (20.328, -22.527) -> (20.055, -21.682)
  line L669 (20.055, -21.682) -> (19.657, -20.639)
  line L670 (19.657, -20.639) -> (19.235, -19.669)
  line L671 (19.235, -19.669) -> (18.713, -18.626)
  line L672 (18.713, -18.626) -> (18.067, -17.532)
  line L673 (18.067, -17.532) -> (17.396, -16.588)
  line L674 (17.396, -16.588) -> (17.42, -16.513)
  line L675 (17.42, -16.513) -> (18.315, -16.513)
  line L676 (24.975, -8.909) -> (25.075, -8.909)
  line L677 (25.075, -8.909) -> (26.789, -9.754)
  line L678 (26.789, -9.754) -> (27.584, -10.077)
  line L679 (27.584, -10.077) -> (27.709, -10.226)
  line L680 (27.709, -10.226) -> (28.355, -11.295)
  line L681 (28.355, -11.295) -> (28.305, -11.469)
  line L682 (28.305, -11.469) -> (26.69, -14.202)
  line L683 (26.69, -14.202) -> (25.919, -15.594)
  line L684 (25.919, -15.594) -> (25.845, -15.668)
  line L685 (25.845, -15.668) -> (25.447, -15.668)
  line L686 (25.447, -15.668) -> (25.398, -15.619)
  line L687 (25.398, -15.619) -> (25.398, -13.879)
  line L688 (25.398, -13.879) -> (25.348, -13.854)
  line L689 (25.348, -13.854) -> (24.677, -13.854)
  line L690 (24.677, -13.854) -> (24.627, -13.904)
  line L691 (24.627, -13.904) -> (24.627, -15.619)
  line L692 (24.627, -15.619) -> (24.578, -15.668)
  line L693 (24.578, -15.668) -> (24.205, -15.668)
  line L694 (24.205, -15.668) -> (24.105, -15.569)
  line L695 (24.105, -15.569) -> (21.67, -11.369)
  line L696 (21.67, -11.369) -> (21.67, -11.295)
  line L697 (21.67, -11.295) -> (22.266, -10.326)
  line L698 (22.266, -10.326) -> (22.465, -10.077)
  line L699 (22.465, -10.077) -> (23.111, -9.829)
  line L700 (23.111, -9.829) -> (24.975, -8.909)
  line L701 (33.648, -16.513) -> (34.468, -16.513)
  line L702 (34.468, -16.513) -> (34.816, -16.588)
  line L703 (34.816, -16.588) -> (34.841, -16.663)
  line L704 (34.841, -16.663) -> (34.319, -17.184)
  line L705 (34.319, -17.184) -> (33.623, -18.029)
  line L706 (33.623, -18.029) -> (33.101, -18.775)
  line L707 (33.101, -18.775) -> (32.455, -19.843)
  line L708 (32.455, -19.843) -> (31.635, -21.558)
  line L709 (31.635, -21.558) -> (30.989, -23.372)
  line L710 (30.989, -23.372) -> (30.741, -24.292)
  line L711 (30.741, -24.292) -> (30.542, -25.236)
  line L712 (30.542, -25.236) -> (30.293, -27.174)
  line L713 (30.293, -27.174) -> (30.268, -28.765)
  line L714 (30.268, -28.765) -> (30.417, -30.38)
  line L715 (30.417, -30.38) -> (30.741, -31.971)
  line L716 (30.741, -31.971) -> (31.188, -33.412)
  line L717 (31.188, -33.412) -> (31.71, -34.679)
  line L718 (31.71, -34.679) -> (32.455, -36.146)
  line L719 (32.455, -36.146) -> (33.499, -37.885)
  line L720 (33.499, -37.885) -> (34.766, -39.749)
  line L721 (34.766, -39.749) -> (36.357, -41.861)
  line L722 (36.357, -41.861) -> (37.848, -43.626)
  line L723 (37.848, -43.626) -> (37.823, -43.7)
  line L724 (37.823, -43.7) -> (36.705, -43.725)
  line L725 (36.705, -43.725) -> (36.605, -43.675)
  line L726 (36.605, -43.675) -> (34.742, -41.315)
  line L727 (34.742, -41.315) -> (33.772, -39.948)
  line L728 (33.772, -39.948) -> (32.753, -38.382)
  line L729 (32.753, -38.382) -> (32.107, -37.264)
  line L730 (32.107, -37.264) -> (31.561, -36.195)
  line L731 (31.561, -36.195) -> (30.865, -34.555)
  line L732 (30.865, -34.555) -> (30.467, -33.412)
  line L733 (30.467, -33.412) -> (30.219, -32.542)
  line L734 (30.219, -32.542) -> (29.995, -31.598)
  line L735 (29.995, -31.598) -> (29.821, -30.629)
  line L736 (29.821, -30.629) -> (29.647, -29.138)
  line L737 (29.647, -29.138) -> (29.622, -27.274)
  line L738 (29.622, -27.274) -> (29.821, -25.261)
  line L739 (29.821, -25.261) -> (30.244, -23.298)
  line L740 (30.244, -23.298) -> (30.517, -22.378)
  line L741 (30.517, -22.378) -> (30.989, -21.061)
  line L742 (30.989, -21.061) -> (31.809, -19.247)
  line L743 (31.809, -19.247) -> (32.306, -18.352)
  line L744 (32.306, -18.352) -> (32.828, -17.532)
  line L745 (32.828, -17.532) -> (33.648, -16.513)
  line L746 (16.377, -16.513) -> (16.998, -17.259)
  line L747 (16.998, -17.259) -> (17.445, -17.905)
  line L748 (17.445, -17.905) -> (18.34, -19.471)
  line L749 (18.34, -19.471) -> (18.738, -20.316)
  line L750 (18.738, -20.316) -> (19.433, -22.105)
  line L751 (19.433, -22.105) -> (19.781, -23.248)
  line L752 (19.781, -23.248) -> (20.055, -24.366)
  line L753 (20.055, -24.366) -> (20.204, -25.186)
  line L754 (20.204, -25.186) -> (20.353, -26.379)
  line L755 (20.353, -26.379) -> (20.403, -27.1)
  line L756 (20.403, -27.1) -> (20.403, -28.914)
  line L757 (20.403, -28.914) -> (20.204, -30.728)
  line L758 (20.204, -30.728) -> (20.005, -31.747)
  line L759 (20.005, -31.747) -> (19.682, -33.014)
  line L760 (19.682, -33.014) -> (19.11, -34.704)
  line L761 (19.11, -34.704) -> (18.415, -36.295)
  line L762 (18.415, -36.295) -> (18.091, -36.941)
  line L763 (18.091, -36.941) -> (17.371, -38.208)
  line L764 (17.371, -38.208) -> (15.855, -40.519)
  line L765 (15.855, -40.519) -> (14.861, -41.861)
  line L766 (14.861, -41.861) -> (13.419, -43.675)
  line L767 (13.419, -43.675) -> (13.345, -43.725)
  line L768 (13.345, -43.725) -> (12.202, -43.7)
  line L769 (12.202, -43.7) -> (12.177, -43.626)
  line L770 (12.177, -43.626) -> (12.873, -42.831)
  line L771 (12.873, -42.831) -> (14.041, -41.389)
  line L772 (14.041, -41.389) -> (15.209, -39.824)
  line L773 (15.209, -39.824) -> (16.725, -37.587)
  line L774 (16.725, -37.587) -> (17.57, -36.17)
  line L775 (17.57, -36.17) -> (18.265, -34.829)
  line L776 (18.265, -34.829) -> (18.912, -33.263)
  line L777 (18.912, -33.263) -> (19.284, -32.045)
  line L778 (19.284, -32.045) -> (19.607, -30.504)
  line L779 (19.607, -30.504) -> (19.756, -28.939)
  line L780 (19.756, -28.939) -> (19.732, -26.976)
  line L781 (19.732, -26.976) -> (19.657, -26.205)
  line L782 (19.657, -26.205) -> (19.483, -25.112)
  line L783 (19.483, -25.112) -> (19.011, -23.223)
  line L784 (19.011, -23.223) -> (18.588, -22.03)
  line L785 (18.588, -22.03) -> (18.265, -21.26)
  line L786 (18.265, -21.26) -> (17.42, -19.57)
  line L787 (17.42, -19.57) -> (17.048, -18.949)
  line L788 (17.048, -18.949) -> (16.327, -17.93)
  line L789 (16.327, -17.93) -> (15.755, -17.234)
  line L790 (15.755, -17.234) -> (15.184, -16.663)
  line L791 (15.184, -16.663) -> (15.209, -16.563)
  line L792 (15.209, -16.563) -> (16.377, -16.513)
  line L793 (24.975, -33.834) -> (25.025, -33.834)
  line L794 (25.025, -33.834) -> (25.099, -33.909)
  line L795 (25.099, -33.909) -> (26.715, -36.643)
  line L796 (26.715, -36.643) -> (26.715, -36.767)
  line L797 (26.715, -36.767) -> (26.541, -37.289)
  line L798 (26.541, -37.289) -> (26.441, -37.488)
  line L799 (26.441, -37.488) -> (26.367, -37.786)
  line L800 (26.367, -37.786) -> (26.118, -38.407)
  line L801 (26.118, -38.407) -> (26.093, -38.556)
  line L802 (26.093, -38.556) -> (25.025, -41.563)
  line L803 (25.025, -41.563) -> (24.95, -41.538)
  line L804 (24.95, -41.538) -> (24.553, -40.345)
  line L805 (24.553, -40.345) -> (24.428, -40.072)
  line L806 (24.428, -40.072) -> (24.031, -38.854)
  line L807 (24.031, -38.854) -> (23.285, -36.792)
  line L808 (23.285, -36.792) -> (23.285, -36.643)
  line L809 (23.285, -36.643) -> (24.627, -34.356)
  line L810 (24.627, -34.356) -> (24.975, -33.834)
  line L811 (19.309, -16.513) -> (23.882, -16.513)
  line L812 (23.882, -16.513) -> (23.956, -16.588)
  line L813 (23.956, -16.588) -> (24.553, -17.607)
  line L814 (24.553, -17.607) -> (24.627, -17.831)
  line L815 (24.627, -17.831) -> (23.683, -19.843)
  line L816 (23.683, -19.843) -> (23.086, -20.987)
  line L817 (23.086, -20.987) -> (23.012, -20.962)
  line L818 (23.012, -20.962) -> (21.297, -18.825)
  line L819 (21.297, -18.825) -> (19.284, -16.588)
  line L820 (19.284, -16.588) -> (19.309, -16.513)
  line L821 (26.938, -20.987) -> (25.422, -17.855)
  line L822 (25.422, -17.855) -> (25.447, -17.681)
  line L823 (25.447, -17.681) -> (25.646, -17.309)
  line L824 (25.646, -17.309) -> (26.168, -16.513)
  line L825 (26.168, -16.513) -> (30.716, -16.513)
  line L826 (30.716, -16.513) -> (30.741, -16.588)
  line L827 (30.741, -16.588) -> (29.001, -18.526)
  line L828 (29.001, -18.526) -> (27.46, -20.365)
  line L829 (27.46, -20.365) -> (27.038, -20.937)
  line L830 (27.038, -20.937) -> (26.938, -20.987)
  line L831 (28.33, -34.158) -> (28.429, -34.207)
  line L832 (28.429, -34.207) -> (28.926, -35.798)
  line L833 (28.926, -35.798) -> (29.771, -38.059)
  line L834 (29.771, -38.059) -> (31.064, -41.166)
  line L835 (31.064, -41.166) -> (32.182, -43.601)
  line L836 (32.182, -43.601) -> (32.182, -43.675)
  line L837 (32.182, -43.675) -> (32.132, -43.725)
  line L838 (32.132, -43.725) -> (31.287, -43.725)
  line L839 (31.287, -43.725) -> (31.138, -43.675)
  line L840 (31.138, -43.675) -> (30.517, -42.259)
  line L841 (30.517, -42.259) -> (29.672, -40.569)
  line L842 (29.672, -40.569) -> (28.131, -37.786)
  line L843 (28.131, -37.786) -> (27.485, -36.692)
  line L844 (27.485, -36.692) -> (27.485, -36.568)
  line L845 (27.485, -36.568) -> (28.33, -34.158)
  line L846 (21.67, -34.207) -> (21.769, -34.406)
  line L847 (21.769, -34.406) -> (22.291, -35.997)
  line L848 (22.291, -35.997) -> (22.465, -36.419)
  line L849 (22.465, -36.419) -> (22.515, -36.667)
  line L850 (22.515, -36.667) -> (20.8, -39.55)
  line L851 (20.8, -39.55) -> (19.98, -41.016)
  line L852 (19.98, -41.016) -> (19.185, -42.607)
  line L853 (19.185, -42.607) -> (18.762, -43.675)
  line L854 (18.762, -43.675) -> (18.688, -43.725)
  line L855 (18.688, -43.725) -> (17.768, -43.725)
  line L856 (17.768, -43.725) -> (17.719, -43.675)
  line L857 (17.719, -43.675) -> (17.744, -43.551)
  line L858 (17.744, -43.551) -> (18.986, -41.016)
  line L859 (18.986, -41.016) -> (20.179, -38.258)
  line L860 (20.179, -38.258) -> (20.949, -36.27)
  line L861 (20.949, -36.27) -> (21.421, -34.878)
  line L862 (21.421, -34.878) -> (21.595, -34.232)
  line L863 (21.595, -34.232) -> (21.67, -34.207)
  line L864 (28.827, -10.624) -> (30.144, -11.17)
  line L865 (30.144, -11.17) -> (33.499, -12.736)
  line L866 (33.499, -12.736) -> (33.499, -12.811)
  line L867 (33.499, -12.811) -> (32.207, -14.55)
  line L868 (32.207, -14.55) -> (31.66, -15.345)
  line L869 (31.66, -15.345) -> (31.561, -15.296)
  line L870 (31.561, -15.296) -> (31.412, -14.998)
  line L871 (31.412, -14.998) -> (29.97, -12.662)
  line L872 (29.97, -12.662) -> (29.15, -11.245)
  line L873 (29.15, -11.245) -> (28.802, -10.698)
  line L874 (28.802, -10.698) -> (28.827, -10.624)
  line L875 (21.173, -10.649) -> (21.198, -10.748)
  line L876 (21.198, -10.748) -> (18.588, -15.072)
  line L877 (18.588, -15.072) -> (18.464, -15.271)
  line L878 (18.464, -15.271) -> (18.365, -15.321)
  line L879 (18.365, -15.321) -> (16.526, -12.811)
  line L880 (16.526, -12.811) -> (16.526, -12.761)
  line L881 (16.526, -12.761) -> (16.998, -12.512)
  line L882 (16.998, -12.512) -> (18.017, -12.065)
  line L883 (18.017, -12.065) -> (18.216, -11.941)
  line L884 (18.216, -11.941) -> (21.098, -10.649)
  line L885 (21.098, -10.649) -> (21.173, -10.649)
  line L886 (19.061, -15.594) -> (21.173, -12.09)
  line L887 (21.173, -12.09) -> (21.272, -12.065)
  line L888 (21.272, -12.065) -> (22.639, -14.351)
  line L889 (22.639, -14.351) -> (23.36, -15.644)
  line L890 (23.36, -15.644) -> (19.085, -15.668)
  line L891 (19.085, -15.668) -> (19.061, -15.594)
  line L892 (26.69, -15.594) -> (28.752, -12.065)
  line L893 (28.752, -12.065) -> (28.827, -12.065)
  line L894 (28.827, -12.065) -> (30.741, -15.196)
  line L895 (30.741, -15.196) -> (30.964, -15.644)
  line L896 (30.964, -15.644) -> (26.715, -15.668)
  line L897 (26.715, -15.668) -> (26.69, -15.594)
  line L898 (25, -18.651) -> (25.05, -18.651)
  line L899 (25.05, -18.651) -> (25.149, -18.8)
  line L900 (25.149, -18.8) -> (26.168, -20.987)
  line L901 (26.168, -20.987) -> (26.491, -21.583)
  line L902 (26.491, -21.583) -> (26.491, -21.682)
  line L903 (26.491, -21.682) -> (25.05, -23.596)
  line L904 (25.05, -23.596) -> (25, -23.596)
  line L905 (25, -23.596) -> (24.876, -23.472)
  line L906 (24.876, -23.472) -> (23.559, -21.658)
  line L907 (23.559, -21.658) -> (23.559, -21.583)
  line L908 (23.559, -21.583) -> (25, -18.651)
  line L909 (26.044, -8.412) -> (26.74, -8.039)
  line L910 (26.74, -8.039) -> (26.914, -7.99)
  line L911 (26.914, -7.99) -> (27.982, -8.487)
  line L912 (27.982, -8.487) -> (29.1, -8.934)
  line L913 (29.1, -8.934) -> (30.666, -9.63)
  line L914 (30.666, -9.63) -> (34.617, -11.245)
  line L915 (34.617, -11.245) -> (34.642, -11.32)
  line L916 (34.642, -11.32) -> (34.071, -12.065)
  line L917 (34.071, -12.065) -> (33.971, -12.065)
  line L918 (33.971, -12.065) -> (31.362, -10.823)
  line L919 (31.362, -10.823) -> (27.063, -8.959)
  line L920 (27.063, -8.959) -> (26.069, -8.487)
  line L921 (26.069, -8.487) -> (26.044, -8.412)
  line L922 (24.006, -8.412) -> (23.981, -8.487)
  line L923 (23.981, -8.487) -> (22.639, -9.133)
  line L924 (22.639, -9.133) -> (19.583, -10.425)
  line L925 (19.583, -10.425) -> (19.483, -10.5)
  line L926 (19.483, -10.5) -> (16.923, -11.643)
  line L927 (16.923, -11.643) -> (16.029, -12.09)
  line L928 (16.029, -12.09) -> (15.954, -12.065)
  line L929 (15.954, -12.065) -> (15.408, -11.344)
  line L930 (15.408, -11.344) -> (15.408, -11.295)
  line L931 (15.408, -11.295) -> (15.507, -11.22)
  line L932 (15.507, -11.22) -> (19.93, -9.431)
  line L933 (19.93, -9.431) -> (20.154, -9.307)
  line L934 (20.154, -9.307) -> (22.565, -8.288)
  line L935 (22.565, -8.288) -> (23.062, -8.039)
  line L936 (23.062, -8.039) -> (23.285, -8.039)
  line L937 (23.285, -8.039) -> (24.006, -8.412)
  line L938 (26.541, -31.3) -> (26.59, -31.3)
  line L939 (26.59, -31.3) -> (27.932, -33.188)
  line L940 (27.932, -33.188) -> (27.932, -33.313)
  line L941 (27.932, -33.313) -> (27.112, -35.698)
  line L942 (27.112, -35.698) -> (27.038, -35.823)
  line L943 (27.038, -35.823) -> (26.963, -35.798)
  line L944 (26.963, -35.798) -> (26.093, -34.282)
  line L945 (26.093, -34.282) -> (25.398, -33.164)
  line L946 (25.398, -33.164) -> (25.77, -32.493)
  line L947 (25.77, -32.493) -> (26.541, -31.3)
  line L948 (23.484, -31.3) -> (24.578, -33.064)
  line L949 (24.578, -33.064) -> (24.602, -33.164)
  line L950 (24.602, -33.164) -> (23.559, -34.853)
  line L951 (23.559, -34.853) -> (23.037, -35.773)
  line L952 (23.037, -35.773) -> (22.937, -35.798)
  line L953 (22.937, -35.798) -> (22.639, -35.002)
  line L954 (22.639, -35.002) -> (22.44, -34.332)
  line L955 (22.44, -34.332) -> (22.316, -34.058)
  line L956 (22.316, -34.058) -> (22.068, -33.313)
  line L957 (22.068, -33.313) -> (22.068, -33.188)
  line L958 (22.068, -33.188) -> (23.41, -31.325)
  line L959 (23.41, -31.325) -> (23.484, -31.3)
  line L960 (36.73, -14.252) -> (36.705, -14.327)
  line L961 (36.705, -14.327) -> (36.108, -14.351)
  line L962 (36.108, -14.351) -> (35.537, -14.476)
  line L963 (35.537, -14.476) -> (34.866, -14.724)
  line L964 (34.866, -14.724) -> (34.195, -15.097)
  line L965 (34.195, -15.097) -> (33.474, -15.668)
  line L966 (33.474, -15.668) -> (32.406, -15.644)
  line L967 (32.406, -15.644) -> (32.43, -15.544)
  line L968 (32.43, -15.544) -> (34.195, -13.109)
  line L969 (34.195, -13.109) -> (34.418, -13.159)
  line L970 (34.418, -13.159) -> (36.73, -14.252)
  line L971 (13.32, -14.252) -> (15.731, -13.109)
  line L972 (15.731, -13.109) -> (15.83, -13.109)
  line L973 (15.83, -13.109) -> (17.644, -15.594)
  line L974 (17.644, -15.594) -> (17.644, -15.644)
  line L975 (17.644, -15.644) -> (16.551, -15.668)
  line L976 (16.551, -15.668) -> (16.153, -15.321)
  line L977 (16.153, -15.321) -> (15.606, -14.948)
  line L978 (15.606, -14.948) -> (15.01, -14.65)
  line L979 (15.01, -14.65) -> (14.314, -14.426)
  line L980 (14.314, -14.426) -> (13.693, -14.327)
  line L981 (13.693, -14.327) -> (13.345, -14.327)
  line L982 (13.345, -14.327) -> (13.32, -14.252)
  line L983 (23.161, -22.378) -> (23.236, -22.378)
  line L984 (23.236, -22.378) -> (24.578, -24.167)
  line L985 (24.578, -24.167) -> (24.578, -24.267)
  line L986 (24.578, -24.267) -> (23.509, -25.733)
  line L987 (23.509, -25.733) -> (23.41, -25.708)
  line L988 (23.41, -25.708) -> (22.266, -24.118)
  line L989 (22.266, -24.118) -> (22.316, -23.944)
  line L990 (22.316, -23.944) -> (23.161, -22.378)
  line L991 (26.864, -22.353) -> (27.758, -24.093)
  line L992 (27.758, -24.093) -> (26.566, -25.733)
  line L993 (26.566, -25.733) -> (26.516, -25.733)
  line L994 (26.516, -25.733) -> (25.497, -24.317)
  line L995 (25.497, -24.317) -> (25.447, -24.192)